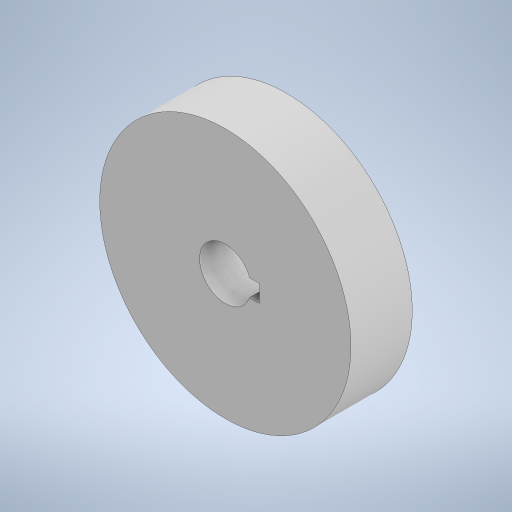
# Autodesk Inventor part: FlanschV2
Saved by Autodesk Inventor 2024.4 (Build 284460000, 460)
## iProperties
Created: 2025-12-02
Part Number: FlanschV2
Material: Generic
Document SubType Name: Modeling
Designer: jonas
Density: 1 g/cm^3
Appearance: Default
Author: jonas
Autodesk Inventor part; units mm, degrees
ref_plane "YZ Plane" through (0, 0, 0) normal (1, 0, 0) x (0, 1, 0)
ref_plane "XZ Plane" through (0, 0, 0) normal (0, 1, 0) x (-1, 0, 0)
ref_plane "XY Plane" through (0, 0, 0) normal (0, 0, 1) x (1, 0, 0)
sketch "Sketch1" plane through (0, 0, 0) normal (0, 1, 0) x (-1, 0, 0)
  arc A0 (-7.1241, -2.5) -> (-7.1241, 2.5) centre (0, 0) ccw
  circle A1 centre (0, 0) radius 36.875
  line L0 (-7.1241, 2.5) -> (-10, 2.5)
  line L1 (-10, 2.5) -> (-10, -2.5)
  line L2 (-10, -2.5) -> (-7.1241, -2.5)
  line L3 (1.186, 0) -> (-1.186, 0) construction
  line L4 (0, -1.583) -> (0, 1.583) construction
  dimension "d0" = 15.1
  dimension "d1" = 73.75
  dimension "d2" = 5
  dimension "d3" = 10
  constraints: 10 end point, 3 coincident, 2 centre point, 2 horizontal, 2 midpoint, 2 point on circle, 1 parallel, 1 perpendicular, 1 vertical, 1 other
  measures "d0" diameter of A0
  measures "d1" diameter of A1
  measures "d2" distance between parallel lines of L2 L0
  measures "d3" distance from line of point (0, 0) L1
extrude "Extrusion1" add sketch "Sketch1" along normal blind 18
body "Solid1"
